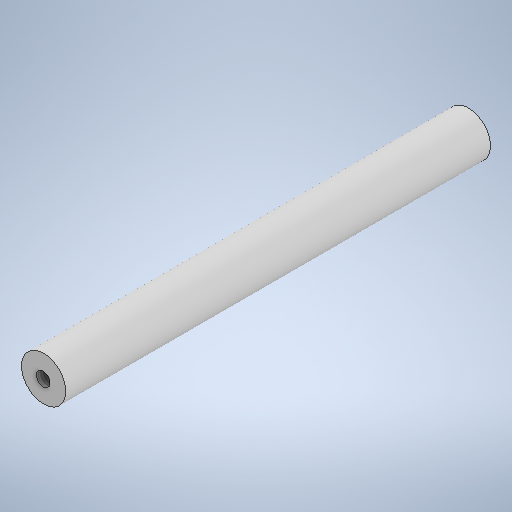
# Autodesk Inventor part: 1886K21_Rotary Shaft _Short
Saved by Autodesk Inventor 2025.1 (Build 291241000, 241)
## iProperties
Company: Managed by Terraform
Created: 2021-09-08
Part Number: 1886K21_Rotary Shaft _Short
Material: Generic
Description: STEP AP203
Document SubType Name: Modeling
Designer: bugme
Density: 1 g/cm^3
Appearance: Default
Sending System: SolidWorks 2017
Preprocessor: SwSTEP 2.0
Title: 1886K21_Rotary Shaft.STEP
Author: Administrator
Revision Number: ANY
Autodesk Inventor part; units mm, degrees
ref_plane "YZ Plane" through (0, 0, 0) normal (1, 0, 0) x (0, 1, 0)
ref_plane "XZ Plane" through (0, 0, 0) normal (0, 1, 0) x (-1, 0, 0)
ref_plane "XY Plane" through (0, 0, 0) normal (0, 0, 1) x (1, 0, 0)
sketch "Sketch3" plane through (0, 0, 0) normal (0, 0, 1) x (1, 0, 0)
  circle A0 centre (0, 0) radius 6.35
  dimension "d0" = 12.7
  constraints: 1 centre point, 1 coincident
  measures "d0" diameter of A0
extrude "Extrusion1" add sketch "Sketch3" along normal mid plane 121.92
sketch "Sketch4" plane through (0, 0, 60.96) normal (0, 0, 1) x (1, 0, 0)
  point P0 (0, 0)
  point P1 (-0.1209, -0.1497)
hole "Hole1" at (-0.1209, -0.1497, 60.96) direction (0, 0, -1) diameter 3.9624 depth 25.4 tip angle 118 thread size "10-32 UNF" class "2B" standard "ANSI Unified Screw Threads"
mirror "Mirror1" about plane through (0, 0, 0) normal (0, 0, 1) of "Hole1"
body "Solid2"
